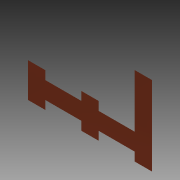
# Autodesk Inventor part: Start_Copper
Saved by Autodesk Inventor 2014 SP1 (Build 180222100, 222)
## iProperties
Created: 2014-01-13
Part Number: Start_Copper
Material: Copper
Document SubType Name: Modeling
Designer: tuleu
Density: 8.94 g/cm^3
Appearance: Copper - Satin
Author: tuleu
Autodesk Inventor part; units mm, degrees
ref_plane "YZ Plane" through (0, 0, 0) normal (1, 0, 0) x (0, 1, 0)
ref_plane "XZ Plane" through (0, 0, 0) normal (0, 1, 0) x (-1, 0, 0)
ref_plane "XY Plane" through (0, 0, 0) normal (0, 0, 1) x (1, 0, 0)
sketch "Sketch1" plane through (0, 0, 0) normal (0, 1, 0) x (-1, 0, 0)
  line L0 (45, -12.5) -> (32.5, -12.5)
  line L1 (32.5, 12.5) -> (45, 12.5)
  line L2 (6.25, -12.5) -> (-6.25, -12.5)
  line L3 (-6.25, 12.5) -> (6.25, 12.5)
  line L4 (-32.5, -12.5) -> (-45, -12.5)
  line L5 (-45, 45) -> (-32.5, 45)
  line L6 (45, 0) -> (-45, 0)
  line L7 (0, -6.25) -> (0, 6.25)
  line L8 (45, 12.5) -> (45, 12.5)
  line L9 (45, 12.5) -> (45, -12.5)
  line L10 (32.5, -12.5) -> (32.5, -6.25)
  line L11 (32.5, 6.25) -> (32.5, 12.5)
  line L12 (32.5, -6.25) -> (6.25, -6.25)
  line L13 (-6.25, -6.25) -> (-32.5, -6.25)
  line L14 (6.25, 12.5) -> (6.25, 6.25)
  line L15 (6.25, -6.25) -> (6.25, -12.5)
  line L16 (-32.5, 6.25) -> (-6.25, 6.25)
  line L17 (6.25, 6.25) -> (32.5, 6.25)
  line L18 (-6.25, -12.5) -> (-6.25, -6.25)
  line L19 (-6.25, 6.25) -> (-6.25, 12.5)
  line L20 (-32.5, 45) -> (-32.5, 6.25)
  line L21 (-32.5, -6.25) -> (-32.5, -12.5)
  line L22 (-45, -12.5) -> (-45, 45)
  line L23 (-45, 12.5) -> (-45, 45)
  point P0 (0, 0)
  dimension "d0" = 12.5
  dimension "d1" = 12.5
  dimension "d2" = 90
  dimension "d3" = 25
  dimension "d4" = 57.5
  constraints: 48 end point, 19 parallel, 10 collinear, 6 perpendicular, 5 horizontal, 5 point on line, 3 midpoint, 5 other
  measures "d0" distance between parallel lines of L17 L12
  measures "d1" distance of L0.start L0.end
  measures "d2" distance between parallel lines of L22 L9
  measures "d3" distance between parallel lines of L1 L0
  measures "d4" distance between parallel lines of L5 L4
extrude "Extrusion1" add sketch "Sketch1" along normal blind 0.01
body "Solid1"
